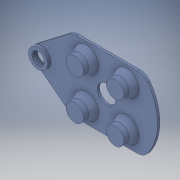
# Autodesk Inventor part: Membrane-DPAD
Saved by Autodesk Inventor 2019 (Build 230136000, 136)
## iProperties
Created: 2019-04-18
Part Number: Membrane-DPAD
Material: Caoutchouc
Document SubType Name: Modeling
Designer: Sébastien DI MERCURIO
Density: 0.93 g/cm^3
Appearance: Caoutchouc - Bleu
Author: Sébastien DI MERCURIO
Autodesk Inventor part; units mm, degrees
ref_plane "YZ Plane" through (0, 0, 0) normal (1, 0, 0) x (0, 1, 0)
ref_plane "XZ Plane" through (0, 0, 0) normal (0, 1, 0) x (-1, 0, 0)
ref_plane "XY Plane" through (0, 0, 0) normal (0, 0, 1) x (1, 0, 0)
sketch "Esquisse1" plane through (0, 0, 0) normal (0, 0, 1) x (1, 0, 0)
  line L0 (-9.1, 11.5) -> (13.9, 11.5)
  circle A0 centre (-19, 0) radius 3.1
  line L1 (-9.1, -11.5) -> (13.9, -11.5)
  line L2 (-9.1, -11.5) -> (-20.8866, -2.4598)
  arc A1 (13.9, -11.5) -> (13.9, 11.5) centre (1.4556, 0) ccw
  circle A2 centre (-19, 0) radius 2
  line L3 (-9.1, 11.5) -> (-20.8866, 2.4598)
  point P0 (0, 0)
  dimension "d0" = 6.2
  dimension "d1" = 23
  dimension "d2" = 23
  dimension "d3" = 23
  dimension "d4" = 11.5
  dimension "d5" = 11.5
  dimension "d6" = 9.9
  dimension "d7" = 9.9
  dimension "d8" = 19
  dimension "d9" = 40.5
  dimension "d10" = 4
  constraints: 8 end point, 4 point on circle, 3 centre point, 2 horizontal, 2 tangent, 1 coincident
  measures "d0" diameter of A0
  measures "d1" distance between parallel lines of L1 L0
  measures "d2" distance of L0.start L0.end
  measures "d3" distance of L1.start L1.end
  measures "d4" distance from line of point (0, 0) L0
  measures "d5" distance from line of L1 A0.centre
  measures "d6" horizontal distance of A0.centre L0.start
  measures "d7" horizontal distance of A0.centre L1.start
  measures "d8" distance of point (0, 0) A0.centre
  measures "d10" diameter of A2
extrude "Extrusion1" add sketch "Esquisse1" along normal blind 0.8
fillet "Congé1" radius 4 2 edges at (13.9, -11.5, 0.4) (13.9, 11.5, 0.4)
fillet "Congé2" radius 4 2 edges at (-9.1, 11.5, 0.4) (-9.1, -11.5, 0.4)
sketch "Esquisse3" plane through (0, 0, 0.8) normal (0, 0, 1) x (1, 0, 0)
  circle A0 centre (-19, 0) radius 2
  circle A1 centre (-19, 0) radius 3.1
  circle A2 centre (-19, 0) radius 2 projected
  point P0 (0, 0)
  dimension "d16" = 4
  dimension "d17" = 6.2
  constraints: 2 centre point, 1 coincident, 1 concentric
  measures "d16" diameter of A0
  measures "d17" diameter of A1
extrude "Extrusion2" add sketch "Esquisse3" along normal blind 1
sketch "Esquisse4" plane through (0, 0, 0.8) normal (0, 0, 1) x (1, 0, 0)
  circle A0 centre (2, 0) radius 3
  line L0 (12.0058, 11.5) -> (-7.7427, 11.5) projected
  circle A1 centre (-19, 0) radius 2 projected
  point P0 (0, 0)
  dimension "d20" = 6
  dimension "d21" = 11.5
  dimension "d22" = 21
  constraints: 1 centre point
  measures "d20" diameter of A0
  measures "d21" distance from line of L0 A0.centre
  measures "d22" distance of A0.centre A1.centre
extrude "Extrusion3" cut sketch "Esquisse4" against normal through all contours A0
sketch "Esquisse5" plane through (0, 0, 0.8) normal (0, 0, 1) x (1, 0, 0)
  circle A0 centre (-4.5, 6.5) radius 4
  circle A1 centre (8.5, 6.5) radius 4
  circle A2 centre (8.5, -6.5) radius 4
  circle A3 centre (-4.5, -6.5) radius 4
  circle A4 centre (2, 0) radius 3 projected
  point P0 (0, 0)
  dimension "d25" = 8
  dimension "d26" = 8
  dimension "d27" = 8
  dimension "d28" = 8
  dimension "d29" = 13
  dimension "d30" = 13
  dimension "d31" = 6.5
  dimension "d32" = 6.5
  dimension "d34" = 6.5
  dimension "d35" = 6.5
  dimension "d36" = 13
  dimension "d37" = 6.5
  constraints: 4 centre point
  measures "d25" diameter of A0
  measures "d26" diameter of A1
  measures "d27" diameter of A3
  measures "d28" diameter of A2
  measures "d29" distance of A1.centre A0.centre
  measures "d30" distance of A2.centre A3.centre
  measures "d31" horizontal distance of A4.centre A0.centre
  measures "d32" horizontal distance of A4.centre A3.centre
  measures "d34" horizontal distance of A1.centre A4.centre
  measures "d35" horizontal distance of A4.centre A2.centre
  measures "d36" distance of A3.centre A0.centre
  measures "d37" horizontal distance of A4.centre A3.centre
extrude "Extrusion4" add sketch "Esquisse5" along normal blind 2 contours A0 | A1 | A2 | A3
sketch "Esquisse7" plane through (-4.5, 6.5, 2.8) normal (0, 0, 1) x (1, 0, 0)
  circle A0 centre (0, 0) radius 2.8
  circle A1 centre (13, 0) radius 2.8
  circle A2 centre (13, -13) radius 2.8
  circle A3 centre (0, -13) radius 2.8
  circle A4 centre (0, 0) radius 4 projected
  circle A5 centre (13, 0) radius 4 projected
  circle A6 centre (13, -13) radius 4 projected
  circle A7 centre (0, -13) radius 4 projected
  point P0 (4.5, -6.5)
  dimension "d49" = 5.6
  dimension "d50" = 5.6
  dimension "d51" = 5.6
  dimension "d52" = 5.6
  constraints: 4 centre point, 4 concentric
  measures "d49" diameter of A0
  measures "d50" diameter of A1
  measures "d51" diameter of A3
  measures "d52" diameter of A2
extrude "Extrusion6" add sketch "Esquisse7" along normal blind 1.7 contours A0 | A1 | A2 | A3
chamfer "Chanfrein2" distance 1.2 distance2 2 1 edges at (-8.5, 6.5, 2.8) measured on face at (-0.9659, 5.9576, 2.8)
chamfer "Chanfrein3" distance 1.2 distance2 2 1 edges at (4.5, 6.5, 2.8) measured on face at (12.0613, 6.1809, 2.8)
chamfer "Chanfrein4" distance 1.2 distance2 2 1 edges at (-8.5, -6.5, 2.8) measured on face at (-0.9659, -7.0424, 2.8)
chamfer "Chanfrein5" distance 1.2 distance2 2 1 edges at (4.5, -6.5, 2.8) measured on face at (12.0341, -7.0424, 2.8)
equation "\"d3\" = d2"
equation "\"d4\" = 0.5 * d1"
equation "\"d5\" = d4"
equation "\"d26\" = d25"
equation "\"d27\" = d25"
equation "\"d28\" = d25"
equation "\"d30\" = d29"
equation "\"d31\" = 0.5 * d29"
equation "\"d32\" = d31"
equation "\"d34\" = d32"
equation "\"d35\" = d32"
equation "\"d36\" = d29"
equation "\"d37\" = d32"
equation "\"d50\" = d49"
equation "\"d51\" = d49"
equation "\"d52\" = d49"
